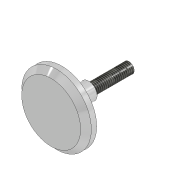
# Autodesk Inventor part: Manija para Bandeja
Saved by Autodesk Inventor 2020 (Build 240168000, 168)
## iProperties
Created: 2020-10-13
Part Number: Manija para Bandeja
Material: Generic
Document SubType Name: Modeling
Designer: Dante
Density: 1 g/cm^3
Appearance: Default
Author: Dante
Autodesk Inventor part; units mm, degrees
ref_plane "YZ Plane" through (0, 0, 0) normal (1, 0, 0) x (0, 1, 0)
ref_plane "XZ Plane" through (0, 0, 0) normal (0, 1, 0) x (-1, 0, 0)
ref_plane "XY Plane" through (0, 0, 0) normal (0, 0, 1) x (1, 0, 0)
sketch "Sketch1" plane through (0, 0, 0) normal (0, 0, 1) x (1, 0, 0)
  circle A0 centre (0, 0) radius 13
  circle A1 centre (0, 0) radius 11.5
  circle A2 centre (0, 0) radius 3.15
  circle A3 centre (0, 0) radius 2
  dimension "d0" = 26
  dimension "d1" = 23
  dimension "d2" = 6.3
  dimension "d3" = 4
  constraints: 4 centre point, 4 coincident
  measures "d0" diameter of A0
  measures "d1" diameter of A1
  measures "d2" diameter of A2
  measures "d3" diameter of A3
extrude "Extrusion1" add sketch "Sketch1" along normal blind 4 contours A0
extrude "Extrusion2" add sketch "Sketch1" along normal blind 4 contours A1 | A2 | A3
extrude "Extrusion3" add sketch "Sketch1" against normal blind 10 contours A2 | A3
extrude "Extrusion4" add sketch "Sketch1" against normal blind 25 contours A3
chamfer "Chamfer1" distance 2 angle 45 1 edges at (-13, 0, 4)
thread "Thread1" size "M4x0.7" class "6g" standard "ISO Metric profile" length 15
body "Solid1"
